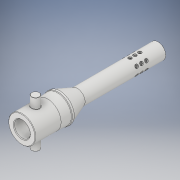
# Autodesk Inventor part: canon
Saved by Autodesk Inventor 2019 (Build 230136000, 136)
## iProperties
Created: 2018-04-17
Part Number: canon
Material: Plastique ABS
Document SubType Name: Modeling
Designer: Theo
Density: 1.06 g/cm^3
Appearance: Lisse - Blanc
Mass: 31.3082 g
Surface Area: 172.508 cm^2
Volume: 29.5361 cm^3
Author: Theo
Autodesk Inventor part; units mm, degrees
ref_plane "YZ Plane" through (0, 0, 0) normal (1, 0, 0) x (0, 1, 0)
sketch "Esquisse1" plane through (0, 0, 0) normal (1, 0, 0) x (0, 1, 0)
  line L0 (13.35, 0) -> (8.775, 0)
  line L1 (8.775, 0) -> (8.15, -0.625)
  line L2 (8.15, -0.625) -> (8.15, -50.15)
  line L3 (13.35, 0) -> (13.85, -0.5)
  line L4 (13.85, -0.5) -> (13.85, -26.5)
  line L5 (8.15, -50.15) -> (6, -50.15)
  line L6 (6, -50.15) -> (6, -105)
  line L7 (6.5, -139.75) -> (6.75, -140)
  line L8 (6.75, -140) -> (7.75, -140)
  line L9 (7.75, -140) -> (8, -139.75)
  line L10 (8, -139.75) -> (8, -57)
  line L11 (6.5, -139.75) -> (6.5, -106)
  line L12 (6, -105) -> (6.5, -106)
  line L13 (14.35, -36.5) -> (13.85, -26.5)
  line L14 (14.35, -36.5) -> (14.85, -37)
  line L15 (14.85, -37) -> (14.85, -39)
  line L16 (14.85, -39) -> (8, -57)
  line L17 (0, 10.3403) -> (0, -80.0023)
  point P0 (0, 0)
  dimension "d4" = 2.15
  dimension "d5" = 0.625
  dimension "d6" = 0.625
  dimension "d7" = 0.5
  dimension "d8" = 0.5
  dimension "d9" = 50.15
  dimension "d11" = 2
  dimension "d12" = 0.25
  dimension "d13" = 0.25
  dimension "d14" = 0.25
  dimension "d15" = 0.25
  dimension "d16" = 34
  dimension "d17" = 0.5
  dimension "d18" = 1
  dimension "d22" = 10
  dimension "d23" = 0.5
  dimension "d27" = 140
  dimension "d43" = 0.5
  dimension "d44" = 0.5
  dimension "d45" = 2
  dimension "d46" = 18
  dimension "d47" = 37
  dimension "d82" = 16.3
  dimension "d83" = 27.7
  dimension "d84" = 12
  constraints: 36 end point, 6 vertical, 3 horizontal, 1 horizontal alignment, 1 point on line
  measures "d4" distance between parallel lines of L6 L2
  measures "d5" horizontal distance of L0.end L1.end
  measures "d6" horizontal distance of L0.end L1.end
  measures "d7" horizontal distance of L0.start L3.end
  measures "d8" horizontal distance of L0.start L3.end
  measures "d9" distance from line of L2.end L0
  measures "d11" distance between parallel lines of L10 L6
  measures "d12" horizontal distance of L8.end L9.end
  measures "d13" horizontal distance of L8.end L9.end
  measures "d14" horizontal distance of L7.start L7.end
  measures "d15" horizontal distance of L7.start L7.end
  measures "d16" distance from line of L11.end L8
  measures "d17" distance from line of L11 L6.end
  measures "d18" vertical distance of L6.end L11.end
  measures "d22" vertical distance of L13.start L4.end
  measures "d23" horizontal distance of L13.start L4.end
  measures "d27" distance between parallel lines of L8 L0
  measures "d43" horizontal distance of L13.start L14.end
  measures "d44" horizontal distance of L13.start L14.end
  measures "d45" distance of L14.end L15.end
  measures "d46" vertical distance of L15.end L10.end
  measures "d47" distance from line of L0 L14.end
  measures "d82" diameter of L2 L17
  measures "d83" diameter of L3.end L17
  measures "d84" diameter of L6 L17
revolve "Révolution1" add sketch "Esquisse1" angle 360 about axis through (0, 0, 10.3403) along (0, 0, -1)
ref_plane "Plan de construction2" through (0, 13.85, -13.5) normal (0, 1, 0) x (-1, 0, 0)
sketch "Esquisse3" plane through (0, 13.85, -13.5) normal (0, 1, 0) x (-1, 0, 0)
  circle A0 centre (0, -0.5) radius 4
  line L0 (0, -154.5) -> (0, 41.5) projected
  line L1 (-13.35, 13.5) -> (13.35, 13.5) projected
  point P0 (0, 13.5)
  dimension "d48" = 8
  dimension "d49" = 14
  constraints: 1 centre point, 1 point on line
  measures "d48" diameter of A0
  measures "d49" distance from line of A0.centre L1
extrude "Extrusion2" add sketch "Esquisse3" along normal blind 10 and the other way blind 2
chamfer "Chanfrein1" distance 0.25 angle 45 4 edges at (4, 13.2598, -14.0006) (-3.043, 13.5116, -11.4038) (-3.043, 13.5116, -16.5962) (4, 23.85, -14)
mirror "Symétrie1" about plane through (0, 0, 0) normal (0, 1, 0) of "Extrusion2", "Chanfrein1"
ref_plane "Plan de construction1" through (0, -8, -98.375) normal (0, 1, 0) x (-1, 0, 0)
sketch "Esquisse5" plane through (0, -8, -98.375) normal (0, 1, 0) x (-1, 0, 0)
  circle A0 centre (0, -22.625) radius 1.5
  circle A1 centre (0, -17.625) radius 1.5
  circle A2 centre (0, -12.625) radius 1.5
  line L0 (-6.5, -7.625) -> (6.5, -7.625) projected
  line L1 (0, -69.625) -> (0, 126.375) projected
  point P0 (0, 98.375)
  dimension "d64" = 5
  dimension "d65" = 3
  dimension "d66" = 5
  dimension "d67" = 5
  constraints: 3 centre point, 3 point on line, 2 equal radius
  measures "d64" distance of A1.centre A0.centre
  measures "d65" diameter of A0
  measures "d66" distance of A2.centre A1.centre
  measures "d67" distance from line of A2.centre L0
extrude "Extrusion3" cut sketch "Esquisse5" along normal up to surface
fillet "Congé2" radius 0.25 12 edges at (1.5, -6.3246, -110.9985) (-1.1294, -7.9199, -110.0128) (1.5, -7.8581, -110.9998) (-1.1286, -7.92, -111.9881) (-1.1294, -7.9199, -115.0128) (1.5, -7.8581, -115.9998) (-1.1286, -7.92, -116.9881) (1.5, -6.3246, -115.9985) (1.5, -6.3246, -120.9985) (-1.1294, -7.9199, -120.0128) (1.5, -7.8581, -120.9998) (-1.1286, -7.92, -121.9881)
pattern_circular "Réseau circulaire3" count 6 over 360 about axis through (0, 0, -10) along (0, 0, 1) of "Extrusion3", "Congé2"
equation "\"d6\" = d5"
equation "\"d8\" = d7"
equation "\"d13\" = d12"
equation "\"d14\" = d12"
equation "\"d15\" = d12"
equation "\"d103\" = 28"
